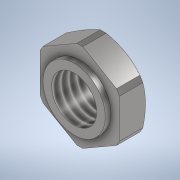
# Autodesk Inventor part: S4-05-3W
Saved by Autodesk Inventor 2020 (Build 240168000, 168)
## iProperties
Part Number: S4-05-3W
Material: チタン
Catalog Web Link: https://jp.misumi-ec.com/vona2/detail/221000555662/?HissuCode=S4-05-3W
Document SubType Name: Modeling
Designer: Masato Kubotera
Density: 8.10141 g/cm^3
Appearance: 半つや出し
Description: ReadyMade
Mass: 0.595 g
Surface Area: 1.55999 cm^2
Volume: 0.073444 cm^3
Author: Masato Kubotera
Autodesk Inventor part; units mm, degrees
ref_plane "YZ Plane" through (0, 0, 0) normal (1, 0, 0) x (0, 1, 0)
ref_plane "XZ Plane" through (0, 0, 0) normal (0, 1, 0) x (-1, 0, 0)
ref_plane "XY Plane" through (0, 0, 0) normal (0, 0, 1) x (1, 0, 0)
sketch "スケッチ1" plane through (0, 0, 0) normal (0, 1, 0) x (-1, 0, 0)
  line L0 (-2, 0) -> (-2, 2.8)
  line L1 (-2, 2.8) -> (-2.75, 2.8)
  line L2 (-2.75, 2.8) -> (-2.75, 2.3)
  line L3 (-2.75, 2.3) -> (-4.0415, 2.3)
  line L4 (-4.0415, 2.3) -> (-4.0415, 0.3126)
  line L5 (-3.5, 0) -> (-2, 0)
  line L6 (-4.0415, 0.3126) -> (-3.5, 0)
  line L7 (0, -0.56) -> (0, 3.36) projected
  point P0 (0, 0)
  dimension "d0" = 3.5
  dimension "d1" = 4.0415
  dimension "d2" = 30
  dimension "d3" = 0.5
  dimension "d4" = 2.8
  dimension "d5" = 4
  dimension "d6" = 5.5
  constraints: 14 end point, 5 perpendicular, 1 point on line, 1 vertical
  measures "d0" distance of L5.start point (0, 0)
  measures "d1" horizontal distance of point (0, 0) L4.end
  measures "d2" angle of L6 L5
  measures "d3" distance of L1.end L2.end
  measures "d4" distance of L0.start L0.end
  measures "d5" diameter of L0 L7
  measures "d6" diameter of L1.end L7
revolve "回転1" add sketch "スケッチ1" angle 360 about axis through (0, 0, -10) along (0, 0, 1)
sketch "スケッチ2" plane through (0, 0, 0) normal (0, 0, -1) x (-1, 0, 0)
  circle A0 centre (0, 0) radius 4.0415 projected
  line L0 (0, 4.0415) -> (3.5, 2.0207)
  line L1 (3.5, 2.0207) -> (3.5, -2.0207)
  line L2 (3.5, -2.0207) -> (0, -4.0415)
  line L3 (0, -4.0415) -> (-3.5, -2.0207)
  line L4 (-3.5, -2.0207) -> (-3.5, 2.0207)
  line L5 (-3.5, 2.0207) -> (0, 4.0415)
  point P0 (-3.5, 2.0207)
  point P1 (-3.5, 2.0207)
  point P2 (-3.5, -2.0207)
  point P3 (-3.5, -2.0207)
  point P4 (0, -4.0415)
  point P5 (0, -4.0415)
  point P6 (3.5, -2.0207)
  point P7 (3.5, -2.0207)
  point P8 (3.5, 2.0207)
  point P9 (3.5, 2.0207)
  constraints: 12 end point, 1 coincident, 1 vertical, 15 other
extrude "押し出し1" cut sketch "スケッチ2" against normal through all contours A0 L1 | L0 A0 | A0 L2 | L5 A0 | A0 L3 | L4 A0
chamfer "面取り1" distance 0.3 angle 45 6 edges at (0, 4.0415, 1.3063) (-3.5, 2.0207, 1.3063) (3.5, 2.0207, 1.3063) (3.5, -2.0207, 1.3063) (0, -4.0415, 1.3063) (-3.5, -2.0207, 1.3063)
thread "ねじ1" size "M4x0.7" class "6H" standard "ANSI Metric M Profile" full length
equation "\"d1\" = 1.1547 * d0"
